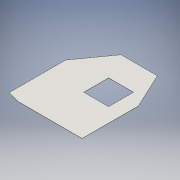
# Autodesk Inventor part: side plate
Saved by Autodesk Inventor 2018 (Build 220112000, 112)
## iProperties
Created: 2018-06-19
Part Number: side plate
Material: Stainless Steel
Document SubType Name: Modeling
Designer: P446509
Density: 8 g/cm^3
Appearance: Steel
Author: P446509
Autodesk Inventor part; units mm, degrees
ref_plane "YZ Plane" through (0, 0, 0) normal (1, 0, 0) x (0, 1, 0)
ref_plane "XZ Plane" through (0, 0, 0) normal (0, 1, 0) x (-1, 0, 0)
ref_plane "XY Plane" through (0, 0, 0) normal (0, 0, 1) x (1, 0, 0)
sketch "Sketch1" plane through (0, 0, 0) normal (0, 0, 1) x (1, 0, 0)
  line L0 (0, 0) -> (-568, 0)
  line L1 (0, 0) -> (0, 496)
  line L2 (0, 0) -> (-147, 0)
  line L3 (-147, 811) -> (0, 496)
  line L4 (-147, 811) -> (-468, 811)
  line L5 (-568, 0) -> (-671.8163, 29.7688)
  line L6 (-568, 0) -> (-460, 0) construction
  line L7 (-671.8163, 29.7688) -> (-671.8163, 525.7688)
  line L8 (-671.8163, 525.7688) -> (-468, 811)
  line L9 (0, 0) -> (-236, 0)
  line L10 (-236, 360) -> (-126, 360)
  line L11 (-126, 360) -> (-126, 580)
  line L12 (-126, 580) -> (-346, 580)
  line L13 (-346, 580) -> (-346, 360)
  line L14 (-346, 360) -> (-236, 360)
  dimension "d0" = 568
  dimension "d1" = 496
  dimension "d2" = 147
  dimension "d3" = 811
  dimension "d4" = 321
  dimension "d5" = 108
  dimension "d6" = 164
  dimension "d7" = 496
  dimension "d8" = 236
  dimension "d9" = 360
  dimension "d10" = 110
  dimension "d11" = 220
  dimension "d12" = 220
  constraints: 30 end point, 4 horizontal, 3 perpendicular, 3 vertical, 2 point on line, 1 equal length
  measures "d0" distance of L0.start L0.end
  measures "d1" distance of L0.start L1.end
  measures "d2" distance of L0.start L2.end
  measures "d3" distance of L2.end L3.start
  measures "d4" distance of L3.start L4.end
  measures "d5" distance of L0.end L5.end
  measures "d6" angle of L6 L5
  measures "d7" distance of L5.end L7.end
  measures "d8" distance of L0.start L9.end
  measures "d9" distance of L9.end L10.start
  measures "d10" distance of L10.start L10.end
  measures "d11" distance of L10.end L11.end
  measures "d12" distance of L11.end L12.end
extrude "Extrusion1" add sketch "Sketch1" along normal blind 1.6
body "Solid1"
